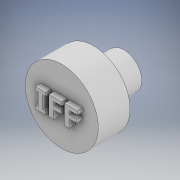
# Autodesk Inventor part: IPC IFF
Saved by Autodesk Inventor 2022 (Build 260153000, 153)
## iProperties
Created: 2022-01-01
Part Number: IPC IFF
Material: Generic
Document SubType Name: Modeling
Designer: solor
Density: 1 g/cm^3
Appearance: Default
Author: solor
Autodesk Inventor part; units mm, degrees
ref_plane "YZ Plane" through (0, 0, 0) normal (1, 0, 0) x (0, 1, 0)
ref_plane "XZ Plane" through (0, 0, 0) normal (0, 1, 0) x (-1, 0, 0)
ref_plane "XY Plane" through (0, 0, 0) normal (0, 0, 1) x (1, 0, 0)
sketch "Sketch1" plane through (0, 0, 0) normal (0, 0, 1) x (1, 0, 0)
  circle A0 centre (0, 0) radius 6.22 construction
  circle A1 centre (0, 0) radius 2.8
  line L0 (-0.675, 0.675) -> (-0.675, 2.025)
  line L1 (-0.675, 2.025) -> (0.675, 2.025)
  line L2 (0.675, 2.025) -> (0.675, 0.675)
  line L3 (0.675, 0.675) -> (2.025, 0.675)
  line L4 (2.025, 0.675) -> (2.025, -0.675)
  line L5 (2.025, -0.675) -> (0.675, -0.675)
  line L6 (0.675, -0.675) -> (0.675, -2.025)
  line L7 (0.675, -2.025) -> (-0.675, -2.025)
  line L8 (-0.675, -2.025) -> (-0.675, -0.675)
  line L9 (-0.675, -0.675) -> (-2.025, -0.675)
  line L10 (-2.025, -0.675) -> (-2.025, 0.675)
  line L11 (-2.025, 0.675) -> (-0.675, 0.675)
  circle A2 centre (0, 0) radius 5.75
  point P0 (-6.07, -6.1)
  dimension "d0" = 12.44
  dimension "d1" = 0.47
  constraints: 24 end point, 3 centre point, 1 coincident
  measures "d0" diameter of A0
  measures "d1" radial gap between concentric circles of A0 A2
extrude "Extrusion1" add sketch "Sketch1" along normal blind 5 contours A1 | L0 L1 L2 L3 L4 L5 L6 L7 L8 L9 L10 L11 | A2
extrude "Extrusion2" add sketch "Sketch1" against normal blind 4.8 contours A1
sketch "Sketch2" plane through (0, 0, 5) normal (0, 0, 1) x (1, 0, 0)
  point P0 (0, 0)
sketch "Sketch3" plane through (0, 0, 5) normal (0, 0, 1) x (1, 0, 0)
  line L0 (-3.4504, 1.525) -> (3.4504, 1.525) construction
  line L1 (3.4504, 1.525) -> (3.4504, -1.525) construction
  line L2 (3.4504, -1.525) -> (-3.4504, -1.525) construction
  line L3 (-3.4504, -1.525) -> (-3.4504, 1.525) construction
  line L4 (-1.6165, -1.525) -> (-3.2576, -1.525)
  line L5 (-3.2576, -1.525) -> (-3.2576, -0.9936)
  line L6 (-3.2576, -0.9936) -> (-2.8201, -0.9936)
  line L7 (-2.8201, -0.9936) -> (-2.8201, 0.9936)
  line L8 (-2.8201, 0.9936) -> (-3.2576, 0.9936)
  line L9 (-3.2576, 0.9936) -> (-3.2576, 1.525)
  line L10 (-3.2576, 1.525) -> (-1.6165, 1.525)
  line L11 (-1.6165, 1.525) -> (-1.6165, 0.9936)
  line L12 (-1.6165, 0.9936) -> (-2.0539, 0.9936)
  line L13 (-2.0539, 0.9936) -> (-2.0539, -0.9936)
  line L14 (-2.0539, -0.9936) -> (-1.6165, -0.9936)
  line L15 (-1.6165, -0.9936) -> (-1.6165, -1.525)
  line L16 (0.9343, 0.9442) -> (-0.346, 0.9442)
  line L17 (-0.346, 0.9442) -> (-0.346, 0.3683)
  line L18 (-0.346, 0.3683) -> (0.8329, 0.3683)
  line L19 (0.8329, 0.3683) -> (0.8329, -0.2126)
  line L20 (0.8329, -0.2126) -> (-0.346, -0.2126)
  line L21 (-0.346, -0.2126) -> (-0.346, -1.525)
  line L22 (-0.346, -1.525) -> (-1.1073, -1.525)
  line L23 (-1.1073, -1.525) -> (-1.1073, 1.525)
  line L24 (-1.1073, 1.525) -> (0.9343, 1.525)
  line L25 (0.9343, 1.525) -> (0.9343, 0.9442)
  line L26 (3.3713, 0.9442) -> (2.091, 0.9442)
  line L27 (2.091, 0.9442) -> (2.091, 0.3683)
  line L28 (2.091, 0.3683) -> (3.27, 0.3683)
  line L29 (3.27, 0.3683) -> (3.27, -0.2126)
  line L30 (3.27, -0.2126) -> (2.091, -0.2126)
  line L31 (2.091, -0.2126) -> (2.091, -1.525)
  line L32 (2.091, -1.525) -> (1.3297, -1.525)
  line L33 (1.3297, -1.525) -> (1.3297, 1.525)
  line L34 (1.3297, 1.525) -> (3.3713, 1.525)
  line L35 (3.3713, 1.525) -> (3.3713, 0.9442)
  point P0 (0, 0)
  point P1 (0, -1.525)
  point P2 (0, 0)
  constraints: 1 midpoint, 2 other
extrude "Extrusion4" add sketch "Sketch3" along normal blind 0.9
body "Solid1"
